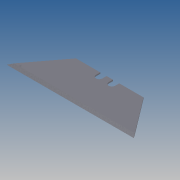
# Autodesk Inventor part: Utility Blade (Stanley)
Saved by Autodesk Inventor 2012 (Build 160160000, 160)
## iProperties
Created: 2015-10-05
Part Number: Utility Blade (Stanley)
Material: Default
Document SubType Name: Modeling
Designer: Lainey
Density: 1 g/cm^3
Author: Lainey
Autodesk Inventor part; units mm, degrees
ref_plane "YZ Plane" through (0, 0, 0) normal (1, 0, 0) x (0, 1, 0)
ref_plane "XZ Plane" through (0, 0, 0) normal (0, 1, 0) x (-1, 0, 0)
ref_plane "XY Plane" through (0, 0, 0) normal (0, 0, 1) x (1, 0, 0)
sketch "Sketch1" plane through (0, 0, 0) normal (0, 0, 1) x (1, 0, 0)
  line L0 (30.125, 0) -> (-30.125, 0)
  line L1 (-16, 18.7) -> (-16, -21.1524) construction
  line L2 (16, 36.5388) -> (16, -18.8821) construction
  line L3 (-16, 18.7) -> (-30.125, 0)
  line L4 (16, 18.7) -> (30.125, 0)
  arc A0 (-4.5, 16.7) -> (-1.5, 16.7) centre (-3, 16.7) ccw
  line L5 (-4.5, 16.7) -> (-4.5, 18.7)
  line L6 (-1.5, 16.7) -> (-1.5, 18.7)
  line L7 (0, 0.7455) -> (0, 23.152) construction
  arc A1 (1.5, 16.7) -> (4.5, 16.7) centre (3, 16.7) ccw
  line L8 (4.5, 16.7) -> (4.5, 18.7)
  line L9 (1.5, 16.7) -> (1.5, 18.7)
  line L10 (4.5, 18.7) -> (16, 18.7)
  line L11 (16, 18.7) -> (4.5, 18.7)
  line L12 (-16, 18.7) -> (-4.5, 18.7)
  line L13 (-1.5, 18.7) -> (1.5, 18.7)
  line L14 (1.5, 18.7) -> (-1.5, 18.7)
  line L15 (-4.5, 18.7) -> (-16, 18.7)
  point P0 (0, 0)
  point P1 (30.125, 18.7)
  point P2 (-30.125, 18.7)
  dimension "d0" = 0
  dimension "d4" = 16
  dimension "d6" = 3
  constraints: 32 end point, 6 perpendicular, 6 symmetric about line, 5 parallel, 4 point on circle, 2 centre point, 2 tangent, 1 horizontal, 1 point on line, 1 other
  measures "d0" distance from line of L0 point (0, 0)
  measures "d4" distance from line of point (0, 0) L2
  measures "d6" diameter of A0
extrude "Extrusion1" add sketch "Sketch1" along normal blind 0.6
chamfer "Chamfer1" distance 0.3 distance2 2 1 edges at (0, 0, 0.6) measured on face at (-10.0417, 0, 0.2)
chamfer "Chamfer2" distance 0.3 distance2 2 1 edges at (0, 0, 0) measured on face at (10.0417, 0, 0.2)
body "Solid1"
